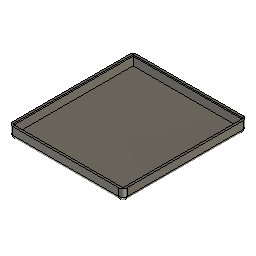
Dragino PCB Case v1 (Autodesk Fusion 360 design; units mm, degrees)
part number: 2026-06-28-10-56-34-278
Autodesk Fusion 360 part; units mm, degrees
sketch "Sketch1" plane through (0, 0, 0) normal (0, 0, 1) x (1, 0, 0)
  line L0 (0, 0) -> (82.25, 0)
  line L1 (82.25, 0) -> (82.25, 89.5)
  line L2 (82.25, 89.5) -> (0, 89.5)
  line L3 (0, 89.5) -> (0, 0)
  dimension "d1" = 89.5
  dimension "d2" = 82.25
  constraint horizontal L0
  constraint vertical L1
  constraint horizontal L2
  constraint vertical L3
  constraint coincident L0.start L3.end
  measures "d1" distance of L0.start L2.end
  measures "d2" distance of L1 L3
extrude "Extrude1" add sketch "Sketch1" along normal blind 8.5
shell "Shell1" thickness 2 removed faces 1 at (27.4167, 59.6667, 8.5)
fillet "Fillet1" radius 3 8 edges at (0, 0, 4.25) (82.25, 0, 4.25) (82.25, 89.5, 4.25) (0, 89.5, 4.25) (41.125, 89.5, 0) (0, 44.75, 0) (41.125, 0, 0) (82.25, 44.75, 0)
chamfer "Chamfer1" distance 0.5 angle 45 4 edges at (2, 44.75, 8.5) (41.125, 2, 8.5) (41.125, 87.5, 8.5) (80.25, 44.75, 8.5)
equation "d1 = 85.5 mm + 4 mm"
equation "d2 = 78.25 mm + 4 mm"
equation "d3 = 6.5 mm + 2 mm"
